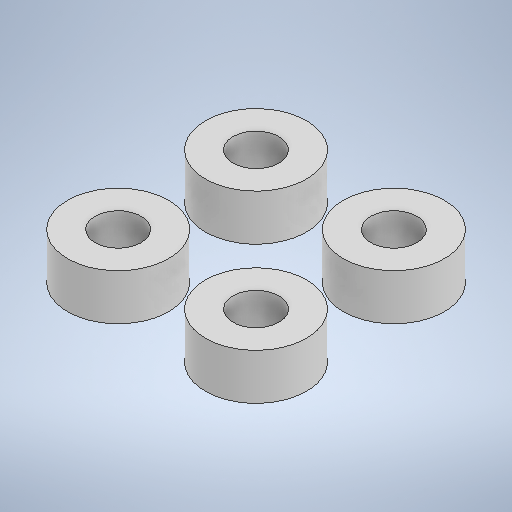
# Autodesk Inventor part: Gripper_Gen3_BearingArray
Saved by Autodesk Inventor 2025.1 (Build 291241000, 241)
## iProperties
Created: 2024-10-29
Part Number: Gripper_Gen3_BearingArray
Material: Generic
Document SubType Name: Modeling
Designer: m_kni
Density: 1 g/cm^3
Appearance: Default
Author: m_kni
Autodesk Inventor part; units mm, degrees
ref_plane "YZ Plane" through (0, 0, 0) normal (1, 0, 0) x (0, 1, 0)
ref_plane "XZ Plane" through (0, 0, 0) normal (0, 1, 0) x (-1, 0, 0)
ref_plane "XY Plane" through (0, 0, 0) normal (0, 0, 1) x (1, 0, 0)
sketch "Sketch1" plane through (0, 0, 0) normal (0, 1, 0) x (-1, 0, 0)
  circle A0 centre (0, 7.5) radius 5.5
  circle A1 centre (0, 7.5) radius 2.5
  line L0 (0, 7.5) -> (7.5, 7.5)
  line L1 (7.5, 7.5) -> (7.5, 0)
  circle A2 centre (15, 7.5) radius 5.5
  circle A3 centre (15, 7.5) radius 2.5
  line L2 (0, 0) -> (7.5, 0)
  circle A4 centre (0, -7.5) radius 5.5
  circle A5 centre (0, -7.5) radius 2.5
  circle A6 centre (15, -7.5) radius 5.5
  circle A7 centre (15, -7.5) radius 2.5
  dimension "d0" = 11
  dimension "d1" = 7.5
  dimension "d2" = 5
  dimension "d3" = 7.5
  constraints: 8 centre point, 6 end point, 6 symmetric about line, 4 coincident, 2 perpendicular, 1 horizontal, 6 other
  measures "d0" diameter of A0
  measures "d1" distance of L2.start A0.centre
  measures "d2" diameter of A1
  measures "d3" distance of L0.start L0.end
extrude "Extrusion1" add sketch "Sketch1" along normal blind 5
body "Solid1"
